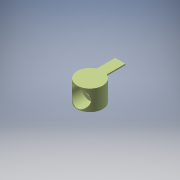
# Autodesk Inventor part: 20-004Z1
Saved by Autodesk Inventor 2018 (Build 220105000, 105)
## iProperties
Created: 2004-10-14
Part Number: 20-004Z1
Material: Zinc ZA-12
Document SubType Name: Modeling
Designer: Autodesk, Inc.
Manufacturer: Standard
Standards Organization: Custom
Description: FASTENER, 40 SERIES, UNIVERSAL
Catalog Web Link: http://www.parker.com/ead/cm1.asp?cmid=809
Vendor: PARKER IPS
Mass: 17.4422 g
Surface Area: 24.0595 cm^2
Volume: 2.88778 cm^3
Density: 6.04 g/cm^3
Appearance: Zinc Chromate 2
CAGE: 1LJX3
Dept. ID: Product Design
Description #2: ---
Finish #1: ---
Finish #2: ---
Material ID: ---
Project Number: ---
Author: Autodesk, Inc.
Autodesk Inventor part; units mm, degrees
ref_plane "YZ Plane" through (0, 0, 0) normal (1, 0, 0) x (0, 1, 0)
ref_plane "XZ Plane" through (0, 0, 0) normal (0, 1, 0) x (-1, 0, 0)
ref_plane "XY Plane" through (0, 0, 0) normal (0, 0, 1) x (1, 0, 0)
sketch "Sketch1" plane through (0, 0, 0) normal (0, 0, 1) x (1, 0, 0)
  circle A0 centre (0, 0) radius 10
  dimension "Diameter" = 20
  constraints: 1 centre point, 1 coincident
  measures "Diameter" diameter of A0
extrude "Base" add sketch "Sketch1" along normal mid plane 16
sketch "Sketch3" plane through (0, 0, 0) normal (0, 1, 0) x (-1, 0, 0)
  line L0 (-10, -8) -> (-10, 8) projected
  line L1 (10, -8) -> (10, 8) projected
  line L2 (-10, 8) -> (10, 8) projected
  line L3 (10, -8) -> (-10, -8) projected
  line L4 (-10, 2.2) -> (0.5164, -8)
  line L5 (-0.5164, -8) -> (10, 2.2)
  line L6 (0, -11.2) -> (0, 11.2) construction
  dimension "d43" = 91.75
  dimension "d44" = 5.8
  constraints: 4 end point, 4 point on line, 1 other
  measures "d43" angle of L5 L4
  measures "d44" distance from line of L2 L4.start
extrude "Pneumatic Cut" [suppressed]
sketch "Sketch2" plane through (0, 0, 8) normal (0, 0, 1) x (1, 0, 0)
  circle A0 centre (0, 0) radius 10 projected
  line L0 (-4, 9.1652) -> (4, 9.1652)
  line L1 (4, 9.1652) -> (4, 23.8)
  line L2 (4, 23.8) -> (-4, 23.8)
  line L3 (-4, 23.8) -> (-4, 9.1652)
  point P0 (0, 23.8)
  dimension "Tab_Length" = 33.8
  dimension "Tab_Width" = 8
  constraints: 8 end point, 2 parallel, 2 point on circle, 1 horizontal, 1 midpoint, 1 perpendicular, 1 vertical alignment
  measures "Tab_Width" distance of L1.end L2.end
extrude "Tab" add sketch "Sketch2" against normal blind 1 contours A0 L3 L2 L1
hole "M6 Thru Hole" [suppressed]
hole "M8 Thru Hole" at (0, -10, 0) direction (0, 1, 0) diameter 9 end through all counterbore diameter 15 counterbore depth 10 clearance for "Socket Head Cap Screw" size "M8" standard "Ansi Metric M Profile"
hole "M6 Threaded" [suppressed]
hole "M8 Threaded" [suppressed]
equation "\"d21\" = 0.5 * Diameter"
equation "\"d8\" = 0.5 * Diameter"
body "Solid1"
